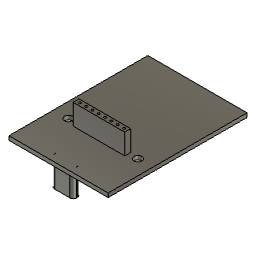
case (Autodesk Fusion 360 archive; units mm, degrees)
design "PCB"
Autodesk Fusion 360 part; units mm, degrees
sketch "Skizze7" plane through (0, 0, 0) normal (0, 0, 1) x (1, 0, 0)
  line L0 (40, 0) -> (40, 56)
  line L1 (0, 0) -> (40, 0)
  line L2 (0, 56) -> (0, 0)
  line L3 (40, 56) -> (0, 56)
  line L4 (19.1939, 4.7) -> (20.8061, 4.7)
  line L5 (20.8061, 1.3) -> (19.1939, 1.3)
  line L6 (24.4922, 4.7) -> (24.4922, 1.3)
  line L7 (15.5, 1.3) -> (15.5, 4.7)
  line L8 (30.4001, 18.6999) -> (9.5999, 18.6999)
  line L9 (30.4001, 16.2998) -> (30.4001, 18.6999)
  line L10 (9.5999, 18.6999) -> (9.5999, 16.2998)
  line L11 (9.5999, 16.2998) -> (30.4001, 16.2998)
  circle A0 centre (34, 18) radius 1.6
  circle A1 centre (6, 18) radius 1.6
  line L12 (15.5, 3) -> (24.4922, 3) construction
  line L13 (20, 4.7) -> (20, 1.3) construction
  line L14 (16.9808, 1.5) -> (23.0114, 1.5)
  arc A2 (23.0114, 1.5) -> (23.0114, 4.5) centre (23.0114, 3) ccw
  line L15 (23.0114, 4.5) -> (16.9808, 4.5)
  arc A3 (16.9808, 4.5) -> (16.9808, 1.5) centre (16.9808, 3) ccw
  line L16 (16.9808, 3) -> (23.0114, 3) construction
  point P0 (19.9961, 3)
  dimension "d25" = 3
  constraint midpoint L7 L12.start
  constraint perpendicular L6 L12
  constraint midpoint L6 L12.end
  constraint midpoint L4 L13.start
  constraint midpoint L5 L13.end
  constraint tangent L14 A2
  constraint tangent A2 L15
  constraint parallel L14 L15
  constraint tangent L15 A3
  constraint tangent L14 A3
  constraint coincident L12 A2.centre
  constraint perpendicular L13 L16
  constraint midpoint L12 P0
  constraint midpoint L16 P0
  measures "d25" diameter of A2
extrude "Extrusion10" add sketch "Skizze7" along normal blind 1.6 contours L0 L1 L2 L3 | L6 L7 L14 A2 L15 A3 | L8 L9 L10 L11
extrude "Extrusion11" add sketch "Skizze7" against normal blind 9.3 contours L6 L7 L14 A2 L15 A3
sketch "Skizze8" plane through (0, 0, 1.6) normal (0, 0, 1) x (-1, 0, 0)
  line L0 (-15.5, -3.2394) -> (-15.5, -2.7606)
  arc A0 (-15.5, -3.2394) -> (-15.5, -2.7606) centre (-16.9808, -3) ccw
  circle A1 centre (-6, -18) radius 1.6
  line L1 (-24.4922, -2.7606) -> (-24.4922, -3.2394)
  arc A2 (-24.4922, -2.7606) -> (-24.4922, -3.2394) centre (-23.0114, -3) ccw
  circle A3 centre (-34, -18) radius 1.6
  line L2 (-40, -56) -> (0, -56)
  line L3 (0, -56) -> (0, 0)
  line L4 (0, 0) -> (-40, 0)
  line L5 (-40, 0) -> (-40, -56)
  line L6 (-9.5999, -16.2998) -> (-30.4001, -16.2998)
  line L7 (-30.4001, -18.6999) -> (-9.5999, -18.6999)
  line L8 (-30.4001, -16.2998) -> (-30.4001, -18.6999)
  line L9 (-9.5999, -18.6999) -> (-9.5999, -16.2998)
extrude "Extrusion12" add sketch "Skizze8" along normal blind 8.3 contours L6 L7 L8 L9
sketch "Skizze9" plane through (0, 0, 9.9) normal (0, 0, 1) x (-1, 0, 0)
  line L0 (-9.5999, -18.6999) -> (-9.5999, -16.2998)
  line L1 (-9.5999, -16.2998) -> (-30.4001, -16.2998)
  line L2 (-30.4001, -16.2998) -> (-30.4001, -18.6999)
  line L3 (-30.4001, -18.6999) -> (-9.5999, -18.6999)
  line L4 (-30.4001, -17.4999) -> (-9.5999, -17.4999) construction
  circle A0 centre (-28.89, -17.4999) radius 0.45
  circle A1 centre (-26.35, -17.4999) radius 0.45
  circle A2 centre (-23.81, -17.4999) radius 0.45
  circle A3 centre (-21.27, -17.4999) radius 0.45
  circle A4 centre (-18.73, -17.4999) radius 0.45
  circle A5 centre (-16.19, -17.4999) radius 0.45
  circle A6 centre (-13.65, -17.4999) radius 0.45
  circle A7 centre (-11.11, -17.4999) radius 0.45
  dimension "d32" = 0.9
  dimension "d35" = 2.54
  dimension "d36" = 0
  dimension "d37" = 1.5101
  dimension "d38" = 1.5101
  constraint midpoint L2 L4.start
  constraint midpoint L0 L4.end
  constraint coincident L4 A0.centre
  measures "d32" diameter of A0
  measures "d37" distance of L2 A0.centre
  measures "d38" distance of L0 A7.centre
extrude "Extrusion13" cut sketch "Skizze9" against normal up to surface (8.3 mm away) contours A0 | A1 | A2 | A3 | A4 | A5 | A6 | A7
equation "d37 = d38"
